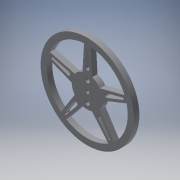
# Autodesk Inventor part: wheel
Saved by Autodesk Inventor 2017.2 (Build 212233000, 233)
## iProperties
Created: 2017-07-13
Part Number: wheel
Material: Generic
Document SubType Name: Modeling
Designer: Nic
Density: 1 g/cm^3
Appearance: Default
Author: Nic
Autodesk Inventor part; units mm, degrees
ref_plane "YZ Plane" through (0, 0, 0) normal (1, 0, 0) x (0, 1, 0)
ref_plane "XZ Plane" through (0, 0, 0) normal (0, 1, 0) x (-1, 0, 0)
ref_plane "XY Plane" through (0, 0, 0) normal (0, 0, 1) x (1, 0, 0)
sketch "Sketch1" plane through (0, 0, 0) normal (0, 1, 0) x (-1, 0, 0)
  circle A0 centre (0, 0) radius 30
  circle A1 centre (0, 0) radius 26
  dimension "d0" = 60
  dimension "d1" = 52
  constraints: 2 centre point, 2 coincident
  measures "d0" diameter of A0
  measures "d1" diameter of A1
extrude "Extrusion1" add sketch "Sketch1" along normal blind 3.5
sketch "Sketch2" plane through (0, 3.5, 0) normal (0, 1, 0) x (1, 0, 0)
  circle A0 centre (0, 0) radius 1.25
  line L0 (0, -27.5) -> (0, 0) construction
  circle A1 centre (0, 0) radius 60 construction
  line L1 (-1.9903, -27.4279) -> (-3.0861, -9.5119)
  line L2 (1.9903, -27.4279) -> (3.0861, -9.5119)
  arc A2 (-0.5773, -24.0366) -> (0.6206, -24.0343) centre (0.0216, -24) ccw
  arc A3 (1.248, -13.0714) -> (-1.2477, -13.0763) centre (0, -13) ccw
  line L3 (-1.2477, -13.0763) -> (-0.5773, -24.0366)
  line L4 (0.6206, -24.0343) -> (1.248, -13.0714)
  line L5 (-2.2, -24) -> (2.2, -24) construction
  line L6 (25.4704, -10.3686) -> (8.0927, -5.8744)
  line L7 (26.7005, -6.5828) -> (10, -0.0042)
  line L8 (23.0497, -6.8368) -> (12.8173, -2.8524)
  arc A4 (12.8173, -2.8524) -> (12.0508, -5.2274) centre (12.3637, -4.0172) ccw
  line L9 (12.0508, -5.2274) -> (22.6818, -7.9768)
  arc A5 (22.6818, -7.9768) -> (23.0497, -6.8368) centre (22.832, -7.3959) ccw
  line L10 (17.7319, 21.0197) -> (8.0877, 5.8813)
  line L11 (14.5115, 23.3595) -> (3.0942, 9.5093)
  line L12 (13.6249, 19.8089) -> (6.6736, 11.3085)
  arc A6 (6.6736, 11.3085) -> (8.6954, 9.8456) centre (7.6412, 10.5172) ccw
  line L13 (8.6954, 9.8456) -> (14.5954, 19.1067)
  arc A7 (14.5954, 19.1067) -> (13.6249, 19.8089) centre (14.0894, 19.4291) ccw
  line L14 (-14.5115, 23.3595) -> (-3.0942, 9.5093)
  line L15 (-17.7319, 21.0197) -> (-8.0877, 5.8813)
  line L16 (-14.6291, 19.0794) -> (-8.6928, 9.8415)
  arc A8 (-8.6928, 9.8415) -> (-6.6767, 11.3123) centre (-7.6412, 10.5172) ccw
  line L17 (-6.6767, 11.3123) -> (-13.6613, 19.7854)
  arc A9 (-13.6613, 19.7854) -> (-14.6291, 19.0794) centre (-14.1243, 19.4037) ccw
  line L18 (-26.7005, -6.5828) -> (-10, -0.0042)
  line L19 (-25.4704, -10.3686) -> (-8.0927, -5.8744)
  line L20 (-22.6662, -8.0172) -> (-12.046, -5.2262)
  arc A10 (-12.046, -5.2262) -> (-12.8219, -2.8542) centre (-12.3637, -4.0172) ccw
  line L21 (-12.8219, -2.8542) -> (-23.0386, -6.8787)
  arc A11 (-23.0386, -6.8787) -> (-22.6662, -8.0172) centre (-22.8187, -7.4369) ccw
  arc A12 (-1.9903, -27.4279) -> (1.9903, -27.4279) centre (0, 0) ccw
  arc A13 (25.4704, -10.3686) -> (26.7005, -6.5828) centre (0, 0) ccw
  arc A14 (17.7319, 21.0197) -> (14.5115, 23.3595) centre (0, 0) ccw
  arc A15 (-14.5115, 23.3595) -> (-17.7319, 21.0197) centre (0, 0) ccw
  arc A16 (-26.7005, -6.5828) -> (-25.4704, -10.3686) centre (0, 0) ccw
  arc A17 (3.0861, -9.5119) -> (8.0927, -5.8744) centre (0, 0) ccw
  arc A18 (10, -0.0042) -> (8.0877, 5.8813) centre (0, 0) ccw
  arc A19 (3.0942, 9.5093) -> (-3.0942, 9.5093) centre (0, 0) ccw
  arc A20 (-8.0877, 5.8813) -> (-10, -0.0042) centre (0, 0) ccw
  arc A21 (-8.0927, -5.8744) -> (-3.0861, -9.5119) centre (0, 0) ccw
  circle A22 centre (0, 0) radius 6.25 construction
  circle A23 centre (0, 6.25) radius 1.5
  circle A24 centre (0, -6.25) radius 1.5
  point P0 (22.1455, -9.5087)
  point P1 (23.5052, -5.3241)
  point P2 (15.8867, 18.1233)
  point P3 (12.327, 20.7095)
  point P4 (-12.327, 20.7095)
  point P5 (-15.8867, 18.1233)
  point P6 (-23.5052, -5.3241)
  point P7 (-22.1455, -9.5087)
  dimension "d11" = 2.5
  dimension "d13" = 120
  dimension "d15" = 3.5
  dimension "d17" = 0.6
  dimension "d18" = 2.5
  dimension "d19" = 24
  dimension "d20" = 13
  dimension "d21" = 0.225
  dimension "d22" = 4.4
  dimension "d25" = 360
  dimension "d27" = 10
  dimension "d28" = 27.5
  dimension "d29" = 12.5
  dimension "d30" = 3
  constraints: 44 end point, 43 point on circle, 25 centre point, 13 point on line, 5 coincident, 4 tangent, 1 equal radius, 1 horizontal, 1 symmetric about line, 1 vertical, 1 vertical alignment, 92 other
  measures "d11" diameter of A0
  measures "d13" diameter of A1
  measures "d15" angle of L1 L0
  measures "d17" radius of A2
  measures "d18" diameter of A3
  measures "d19" distance of L0.end A2.centre
  measures "d20" distance of point (0, 0) A3.centre
  measures "d21" angle of L4 L2
  measures "d22" distance of L5.start L5.end
  measures "d27" radius of A17
  measures "d28" radius of A12
  measures "d29" diameter of A22
  measures "d30" diameter of A24
extrude "Extrusion2" add sketch "Sketch2" against normal up to surface (3.5 mm away)
body "Solid1"
